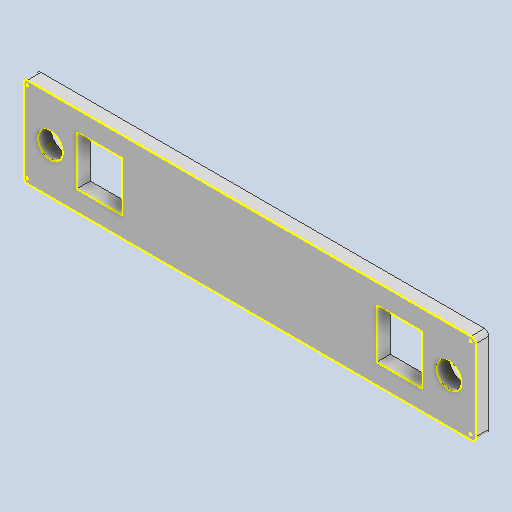
# Autodesk Inventor part: LED_Holder_BackTop
Saved by Autodesk Inventor 2022 (Build 260153000, 153)
## iProperties
Created: 2021-02-24
Part Number: LED_Holder_BackTop
Material: Generic
Document SubType Name: Modeling
Designer: Viktor
Density: 1 g/cm^3
Appearance: Default
Author: Viktor
Autodesk Inventor part; units mm, degrees
ref_plane "YZ Plane" through (0, 0, 0) normal (1, 0, 0) x (0, 1, 0)
ref_plane "XZ Plane" through (0, 0, 0) normal (0, 1, 0) x (-1, 0, 0)
ref_plane "XY Plane" through (0, 0, 0) normal (0, 0, 1) x (1, 0, 0)
sketch "Sketch1" plane through (0, 0, 0) normal (0, 0, 1) x (1, 0, 0)
  line L0 (-95, -10) -> (95, -10)
  line L1 (95, -10) -> (95, 10)
  line L2 (95, 10) -> (-95, 10)
  line L3 (-95, 10) -> (-95, -10)
  line L4 (-95, -10) -> (95, 10) construction
  line L5 (95, -10) -> (-95, 10) construction
  line L6 (-133, 0) -> (133, 0) construction
  line L7 (-83, -5.5) -> (-6, -5.5)
  line L8 (-6, -5.5) -> (-6, 5.5)
  line L9 (-6, 5.5) -> (-83, 5.5)
  line L10 (-83, 5.5) -> (-83, -5.5)
  line L11 (-83, -5.5) -> (-6, 5.5) construction
  line L12 (-6, -5.5) -> (-83, 5.5) construction
  line L13 (0, 14.2899) -> (0, -14.2899) construction
  line L14 (83, -5.5) -> (6, -5.5)
  line L15 (6, -5.5) -> (6, 5.5)
  line L16 (6, 5.5) -> (83, 5.5)
  line L17 (83, 5.5) -> (83, -5.5)
  line L18 (83, -5.5) -> (6, 5.5) construction
  line L19 (6, -5.5) -> (83, 5.5) construction
  circle A0 centre (-89, 0) radius 2.75
  circle A1 centre (0, 0) radius 2.75
  circle A2 centre (89, 0) radius 2.75
  line L20 (-83, 5.5) -> (-73, 5.5)
  line L21 (-73, 5.5) -> (-73, -5.5)
  line L22 (-73, -5.5) -> (-83, -5.5)
  line L23 (-83, -5.5) -> (-83, 5.5)
  line L24 (-6, 5.5) -> (-16, 5.5)
  line L25 (-16, 5.5) -> (-16, -5.5)
  line L26 (-16, -5.5) -> (-6, -5.5)
  line L27 (-6, -5.5) -> (-6, 5.5)
  line L28 (16, 5.5) -> (16, -5.5)
  line L29 (73, 5.5) -> (73, -5.5)
  line L30 (6, 10) -> (6, 5.4904)
  line L31 (6, 5.4904) -> (6, -10)
  point P0 (-44.5, 0)
  point P1 (44.5, 0)
  point P2 (73, -5.5)
  point P3 (73, 5.5)
  point P4 (-73, 5.5)
  point P5 (6, -5.5)
  dimension "d0" = 190
  dimension "d1" = 20
  dimension "d2" = 11
  dimension "d3" = 12
  dimension "d4" = 6
  dimension "d5" = 5.5
  dimension "d6" = 6
  dimension "d7" = 5.5
  dimension "d11" = 10
  dimension "d12" = 10
  constraints: 60 end point, 10 symmetric about line, 8 parallel, 8 point on line, 6 midpoint, 4 horizontal, 4 perpendicular, 3 centre point, 1 coincident, 1 vertical, 1 other
  measures "d0" distance between parallel lines of L1 L3
  measures "d1" distance between parallel lines of L0 L2
  measures "d2" distance between parallel lines of L7 L9
  measures "d3" distance between parallel lines of L3 L10
  measures "d4" horizontal distance of point (0, 0) L8.end
  measures "d5" diameter of A0
  measures "d6" distance from line of L10 A0.centre
  measures "d7" diameter of A1
  measures "d11" distance between parallel lines of L10 L21
  measures "d12" distance between parallel lines of L8 L25
extrude "Extrusion1" add sketch "Sketch1" along normal blind 3 contours L3 L2 L30 L15 L31 L0 | L21 L9 L25 L7
fillet "Fillet1" radius 1 4 edges at (-95, -10, 1.5) (-95, 10, 1.5) (6, 10, 1.5) (6, -10, 1.5)
sketch "Sketch2" plane through (0, 0, 3) normal (0, 0, 1) x (1, 0, 0)
  line L0 (-16, 5.5) -> (-6, 5.5) projected
  line L1 (-6, 5.5) -> (-6, -5.5) projected
  line L2 (-6, -5.5) -> (-16, -5.5) projected
  line L3 (-16, -5.5) -> (-16, 5.5) projected
  circle A0 centre (-89, 0) radius 2.75 projected
  circle A1 centre (0, 0) radius 2.75 projected
  arc A2 (5, -10) -> (6, -9) centre (5, -9) ccw projected
  line L4 (6, -9) -> (6, 9) projected
  arc A3 (6, 9) -> (5, 10) centre (5, 9) ccw projected
  line L5 (5, 10) -> (-94, 10) projected
  arc A4 (-94, 10) -> (-95, 9) centre (-94, 9) ccw projected
  line L6 (-95, 9) -> (-95, -9) projected
  arc A5 (-95, -9) -> (-94, -10) centre (-94, -9) ccw projected
  line L7 (-94, -10) -> (5, -10) projected
  line L8 (-73, 5.5) -> (-73, -5.5) projected
  line L9 (-73, -5.5) -> (-83, -5.5) projected
  line L10 (-83, -5.5) -> (-83, 5.5) projected
  line L11 (-83, 5.5) -> (-73, 5.5) projected
equation "\"d6\" = 0.5 * d3"
equation "\"d7\" = d5"
equation "\"d12\" = d11"
body "Solid1"
